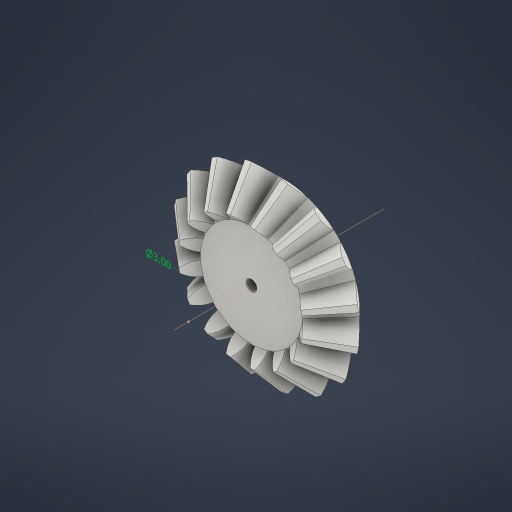
# Autodesk Inventor part: Bevel Gear2
Saved by Autodesk Inventor 2024 (Build 280153000, 153)
## iProperties
CustomPartVersion: 1
Created: 2024-03-09
Part Number: Bevel Gear2
Material: Steel, Mild
Document SubType Name: Modeling
Designer: LightStore
Categories: <?xml version="1.0" encoding="UTF-16"?> <MemberInstance><Categories><FamilyTemplate><FamilyTemplateParameter ValueType="xs:double" Id="1" ObjectReferenceKey="da_z" ObjectType="kUserParameterObject"/><FamilyTemplateParameter ValueType="xs:double" Id="2" ObjectReferenceKey="da_b" ObjectType="kUserParameterObject"/><FamilyTemplateParameter ValueType="xs:double" Id="3" ObjectReferenceKey="da_beta" ObjectType="kUserParameterObject"/><FamilyTemplateParameter ValueType="xs:double" Id="4" ObjectReferenceKey="da_dae" ObjectType="kUserParameterObject"/><FamilyTemplateParameter ValueType="xs:double" Id="5" ObjectReferenceKey="da_ve" ObjectType="kUserParameterObject"/><FamilyTemplateParameter ValueType="xs:double" Id="6" ObjectReferenceKey="da_omega" ObjectType="kUserParameterObject"/><FamilyTemplateParameter ValueType="xs:string" Id="7" ObjectReferenceKey="EAIAABAAAAAAHwAAAAAAAIAAAAAAAAAA" ObjectType="83914240" SubObjectId="SurfaceGeometry"/></FamilyTemplate><ParamToTemplateMap><ParamToTemplate CategoryParameter="//CategoryParameter[@InternalName='046C89C9-8512-4d59-83FE-43B91F4F132A']" TemplateParameter="1"/><ParamToTemplate CategoryParameter="//CategoryParameter[@InternalName='2552DF32-E462-4b46-AEBF-C6C7768E72AC']" TemplateParameter="2"/><ParamToTemplate CategoryParameter="//CategoryParameter[@InternalName='C9EE641D-15FC-4fae-A226-E94C4372FDD7']" TemplateParameter="3"/><ParamToTemplate><ParamToTemplate CategoryParameter="//CategoryParameter[@InternalName='00B6519A-459B-49c7-AD84-2E56D39A5744']" ConstantValue="-0.000000"/></ParamToTemplate><ParamToTemplate><ParamToTemplate CategoryParameter="//CategoryParameter[@InternalName='04B31F0E-C7A6-4894-AA32-9629BEFACF47']" ConstantValue="1.000000"/></ParamToTemplate><ParamToTemplate><ParamToTemplate CategoryParameter="//CategoryParameter[@InternalName='43CBEC2E-7847-49e7-A936-2F7889FCB2D9']" ConstantValue="0.200000"/></ParamToTemplate><ParamToTemplate><ParamToTemplate CategoryParameter="//CategoryParameter[@InternalName='B1EFC894-105D-4ebd-86BF-FA20ED196853']" ConstantValue="0.300000"/></ParamToTemplate><ParamToTemplate><ParamToTemplate CategoryParameter="//CategoryParameter[@InternalName='51175063-3D10-4879-93E8-6246FE8B403D']" ConstantValue="2060000000.000000"/></ParamToTemplate><ParamToTemplate><ParamToTemplate CategoryParameter="//CategoryParameter[@InternalName='A3A52E27-4454-46a9-B0BD-C932399B70AF']" ConstantValue="0.300000"/></ParamToTemplate><ParamToTemplate CategoryParameter="//CategoryParameter[@InternalName='2A200944-5A8C-41ca-B96E-8520D2E510F1']" TemplateParameter="4"/><ParamToTemplate><ParamToTemplate CategoryParameter="//CategoryParameter[@InternalName='1A637F62-92C8-44bc-B81F-10802510B579']" ConstantValue="3.484953"/></ParamToTemplate><ParamToTemplate CategoryParameter="//CategoryParameter[@InternalName='B52DD4BE-6863-48fb-BF58-89EF6F9EC65C']" TemplateParameter="5"/><ParamToTemplate><ParamToTemplate CategoryParameter="//CategoryParameter[@InternalName='3956BFF2-84D2-457d-93C2-9B0613DEBA67']" ConstantValue="1.459462"/></ParamToTemplate><ParamToTemplate CategoryParameter="//CategoryParameter[@InternalName='739CFA02-461B-4bf8-8049-181FCAD8B28F']" TemplateParameter="6"/><ParamToTemplate><ParamToTemplate CategoryParameter="//CategoryParameter[@InternalName='A27E999F-E2CE-4481-8A2A-EBF499C4C3C5']" ConstantValue="-0.000000"/></ParamToTemplate><ParamToTemplate><ParamToTemplate CategoryParameter="//CategoryParameter[@InternalName='9E1B4470-B2D3-4ff1-B813-535BB4CDF51A']" ConstantValue="3520000.000000"/></ParamToTemplate><ParamToTemplate><ParamToTemplate CategoryParameter="//CategoryParameter[@InternalName='F8452263-BFF6-458c-9FB1-07C4B99E95CD']" ConstantValue="11400000.000000"/></ParamToTemplate><ParamToTemplate><ParamToTemplate CategoryParameter="//CategoryParameter[@InternalName='3E3BB259-FD49-497f-8171-6EBC954A3479']" ConstantValue="2.000000"/></ParamToTemplate><ParamToTemplate CategoryParameter="//CategoryParameter[@InternalName='27C3BAF2-7550-4e4b-AE2C-0DB134B7D9B7']" TemplateParameter="7"/></ParamToTemplateMap><Category DisplayName="Gear" InternalName="DC85795E-93AB-48d5-8EEE-5A27447B64BD" Mnemonic="Gear"><CategoryParameter DisplayName="z" InternalName="046C89C9-8512-4d59-83FE-43B91F4F132A" Mnemonic="z"/><CategoryParameter DisplayName="b" InternalName="2552DF32-E462-4b46-AEBF-C6C7768E72AC" Mnemonic="b"/><CategoryParameter DisplayName="||b|" InternalName="C9EE641D-15FC-4fae-A226-E94C4372FDD7" Mnemonic="beta"/><CategoryParameter DisplayName="x" InternalName="00B6519A-459B-49c7-AD84-2E56D39A5744" Mnemonic="x"/><CategoryParameter DisplayName="a*" InternalName="04B31F0E-C7A6-4894-AA32-9629BEFACF47" Mnemonic="a"/><CategoryParameter DisplayName="c*" InternalName="43CBEC2E-7847-49e7-A936-2F7889FCB2D9" Mnemonic="c"/><CategoryParameter DisplayName="r|.f|*" InternalName="B1EFC894-105D-4ebd-86BF-FA20ED196853" Mnemonic="rf"/><CategoryParameter DisplayName="E" InternalName="51175063-3D10-4879-93E8-6246FE8B403D" Mnemonic="E"/><CategoryParameter DisplayName="||m|" InternalName="A3A52E27-4454-46a9-B0BD-C932399B70AF" Mnemonic="mi"/><Category DisplayName="BevelGear" InternalName="0C98F69A-0C2B-4791-B2FE-7691BB227E77" Mnemonic="BevelGear"><CategoryParameter DisplayName="d|.ae|" InternalName="2A200944-5A8C-41ca-B96E-8520D2E510F1" Mnemonic="dae"/><CategoryParameter DisplayName="d|.ai|" InternalName="1A637F62-92C8-44bc-B81F-10802510B579" Mnemonic="dai"/><CategoryParameter DisplayName="A|.e|" InternalName="B52DD4BE-6863-48fb-BF58-89EF6F9EC65C" Mnemonic="ve"/><CategoryParameter DisplayName="A|.i|" InternalName="3956BFF2-84D2-457d-93C2-9B0613DEBA67" Mnemonic="vi"/><CategoryParameter DisplayName="||S|" InternalName="739CFA02-461B-4bf8-8049-181FCAD8B28F" Mnemonic="omega"/><CategoryParameter DisplayName="x|.t|" InternalName="A27E999F-E2CE-4481-8A2A-EBF499C4C3C5" Mnemonic="xt"/><CategoryParameter DisplayName="||s||.Flim|" InternalName="9E1B4470-B2D3-4ff1-B813-535BB4CDF51A" Mnemonic="sFlim"/><CategoryParameter DisplayName="||s||.Hlim|" InternalName="F8452263-BFF6-458c-9FB1-07C4B99E95CD" Mnemonic="sHlim"/><CategoryParameter DisplayName="type" InternalName="3E3BB259-FD49-497f-8171-6EBC954A3479" Mnemonic="type"/><CategoryParameter DisplayName="PitchDiameter" InternalName="27C3BAF2-7550-4e4b-AE2C-0DB134B7D9B7" Mnemonic="IDS_PITCHDIAM"/></Category></Category></Categories></MemberInstance>
Mass: 60.9118 g
Surface Area: 34.3074 cm^2
Volume: 7.7496 cm^3
Density: 7.86 g/cm^3
Appearance: Steel
Author: LightStore
Autodesk Inventor part; units mm, degrees
ref_plane "Mesh Plane2" through (0, 0, 0) normal (0.9807853, 0.1950903, 0) x (0, 0, 1)
sketch "Teeth Body Sketch" plane through (0, 0, 0) normal (1, 0, 0) x (0, 1, 0)
  line L0 (0, 0) -> (21.454416, -26.545584) construction
  line L1 (21.454416, -26.545584) -> (26.12132, -21.87868)
  line L2 (26.12132, -21.87868) -> (0, 0) construction
  line L3 (24, -24) -> (0, 0) construction
  line L4 (14.311609, -17.707778) -> (17.424764, -14.594623)
  line L5 (21.454416, -26.545584) -> (14.311609, -17.707778)
  line L6 (26.12132, -21.87868) -> (17.424764, -14.594623)
  line L7 (0, -39.386751) -> (0, 6.564458)
  line L8 (0, -24) -> (26.12132, -24) construction
  dimension "d0" = 48
  dimension "d1" = 42.90883
  dimension "d2" = 52.24264
  dimension "d3" = 11.3
  dimension "d4" = 21.87868
  constraints: 16 end point, 4 point on line, 3 perpendicular, 2 collinear, 1 horizontal alignment, 1 vertical alignment
  measures "d0" diameter of L3.start L7
  measures "d1" diameter of L0.end L7
  measures "d2" diameter of L1.end L7
  measures "d3" distance between parallel lines of L1 L4
  measures "d4" vertical distance of L1.end L0.start
revolve "Teeth Body" add sketch "Teeth Body Sketch" angle 360 about axis through (0, 0, 0) along (0, 0, 1)
ref_plane "Tooth Plane" through (0, 24, -24) normal (0, -0.7071068, 0.7071068) x (1, 0, 0)
sketch "Start Sketch" plane through (0, 24, -24) normal (0, -0.7071068, 0.7071068) x (1, 0, 0)
  line L0 (0, -23.505131) -> (0, 10.644758)
  arc A0 (-1.269242, -4.392) -> (-5.97451, 4.518714) centre (-13.855964, -5.340713) ccw
  arc A1 (5.97451, 4.518714) -> (1.269242, -4.392) centre (13.855964, -5.340713) ccw
  line L1 (-1.269242, -4.392) -> (1.269242, -4.392)
  arc A2 (5.97451, 4.518714) -> (-5.97451, 4.518714) centre (0, -33.941125) ccw
  dimension "d7" = 12.62242
  dimension "d8" = 13.85596
  dimension "d9" = 28.60041
  dimension "d57" = 38.92113
  dimension "d58" = 29.54913
  constraints: 6 point on circle, 3 centre point, 3 symmetric about line, 2 end point, 1 coincident, 1 perpendicular, 1 other
  measures "d7" radius of A0
  measures "d8" horizontal distance of point (0, -33.941) A0.centre
  measures "d9" vertical distance of point (0, -33.941) A0.centre
  measures "d57" radius of A2
  measures "d58" distance from line of A2.centre L1
sketch "End Sketch" plane through (0, 15.776348, -15.776348) normal (0, -0.7071068, 0.7071068) x (1, 0, 0)
  line L0 (0, -15.35404) -> (0, 6.953444)
  arc A0 (-0.834334, -2.887072) -> (-3.927331, 2.970367) centre (-9.108188, -3.510706) ccw
  arc A1 (3.927331, 2.970367) -> (0.834334, -2.887072) centre (9.108188, -3.510706) ccw
  line L1 (-0.834334, -2.887072) -> (0.834334, -2.887072)
  arc A2 (3.927331, 2.970367) -> (-3.927331, 2.970367) centre (0, -22.311125) ccw
  dimension "d12" = 8.29732
  dimension "d15" = 9.10819
  dimension "d16" = 18.80042
  dimension "d59" = 25.58472
  dimension "d60" = 19.42405
  constraints: 6 point on circle, 3 centre point, 3 symmetric about line, 2 end point, 1 coincident, 1 other
  measures "d12" radius of A0
  measures "d15" horizontal distance of A0.centre point (0, -22.311)
  measures "d16" vertical distance of A0.centre point (0, -22.311)
  measures "d59" radius of A2
  measures "d60" distance from line of A2.centre L1
loft "Loft" cut profiles "Start Sketch", "End Sketch"
pattern_circular "Circular Pattern" count 16 over 360 about axis through (0, 0, 0) along (0, 0, 1) of "Loft"
ref_plane "End Plane" through (0, 15.776348, -15.776348) normal (0, -0.7071068, 0.7071068) x (1, 0, 0)
sketch3d "3D Sketch Right"
ref_plane "End Plane Right" through (-3.313379, 15.424483, -15.776348) normal (0.1485079, -0.6913359, 0.7071068) x (0.9776967, 0.210022, 0)
sketch "End Sketch Right" plane through (-3.313379, 15.424483, -15.776348) normal (0.1485079, -0.6913359, 0.7071068) x (0.9776967, 0.210022, 0)
  arc A0 (-0.834334, -2.887072) -> (-3.927331, 2.970367) centre (-9.108188, -3.510706) ccw
  line L0 (0, -30.205233) -> (0, 11.660762)
  arc A1 (3.927331, 2.970367) -> (0.834334, -2.887072) centre (9.108188, -3.510706) ccw
  line L1 (-0.834334, -2.887072) -> (0.834334, -2.887072)
  arc A2 (3.927331, 2.970367) -> (-3.927331, 2.970367) centre (0, -22.311125) ccw
  dimension "d70" = 9.10819
  dimension "d71" = 18.80042
  dimension "d72" = 8.29732
  dimension "d73" = 19.42405
  dimension "d74" = 25.58472
  constraints: 6 point on circle, 3 centre point, 3 symmetric about line, 2 end point, 1 coincident, 1 perpendicular, 1 other
  measures "d70" horizontal distance of A2.centre A0.centre
  measures "d71" vertical distance of point (0, -22.311) A0.centre
  measures "d72" radius of A0
  measures "d73" distance from line of point (0, -22.311) L1
  measures "d74" radius of A2
feature "Loft Right" [suppressed]
pattern_circular "Circular Pattern Right" [suppressed]
sketch3d "3D Sketch Left"
ref_plane "End Plane Left" through (3.335768, 15.424483, -15.785404) normal (-0.1494462, -0.6910343, 0.707204) x (0.9774044, -0.2113779, 0)
sketch "End Sketch Left" plane through (3.335768, 15.424483, -15.785404) normal (-0.1494462, -0.6910343, 0.707204) x (0.9774044, -0.2113779, 0)
  line L0 (0, -32.902845) -> (0, 14.363747)
  arc A0 (-0.834334, -2.884005) -> (-3.927331, 2.973434) centre (-9.108188, -3.507639) ccw
  arc A1 (3.927331, 2.973434) -> (0.834334, -2.884005) centre (9.108188, -3.507639) ccw
  line L1 (-0.834334, -2.884005) -> (0.834334, -2.884005)
  ellipse E0 centre (0, -10.318538) end of major axis (17.424764, -10.318538) minor radius 12.322862
  arc A2 (3.927331, 2.973434) -> (-3.927331, 2.973434) centre (0, -22.308059) ccw
  dimension "d56" = 12.32286
  dimension "d30" = 8.29732
  dimension "d31" = 9.10819
  dimension "d32" = 18.80042
  dimension "d61" = 25.58472
  dimension "d62" = 19.42405
  constraints: 6 point on circle, 3 centre point, 3 symmetric about line, 2 end point, 1 coincident, 2 other
  measures "d30" radius of A0
  measures "d31" horizontal distance of point (0, -22.308) A0.centre
  measures "d32" vertical distance of A0.centre point (0, -22.308)
  measures "d61" radius of A2
  measures "d62" distance from line of point (0, -22.308) L1
feature "Loft Left" [suppressed]
pattern_circular "Circular Pattern Left" [suppressed]
sketch "Body Sketch" plane through (0, 0, 0) normal (1, 0, 0) x (0, 1, 0)
  line L0 (0, -35.037536) -> (0, -19.530831)
  line L1 (21.454416, -26.545584) -> (14.311609, -17.707778)
  line L2 (14.311609, -17.707778) -> (0, -17.707778)
  line L3 (21.454416, -26.545584) -> (0, -26.545584)
  constraints: 4 end point, 2 perpendicular, 2 point on line
sketch "Body Sketch outline for Fix Body" plane through (0, 0, 0) normal (1, 0, 0) x (0, 1, 0)
  line L0 (0, -26.545584) -> (21.454416, -26.545584)
  line L1 (0, -17.707778) -> (0, -26.545584)
  line L2 (14.311609, -17.707778) -> (0, -17.707778)
  line L3 (21.454416, -26.545584) -> (14.311609, -17.707778)
revolve "Fix Body" add sketch "Body Sketch outline for Fix Body" angle 360 about axis through (0, 0, 0) along (0, 0, 1)
sketch "Sketch6" plane through (0, 0, 0) normal (1, 0, 0) x (0, 1, 0)
  line L0 (24, -24) -> (0, 0)
  line L1 (0, -37.799919) -> (0, 6.299986)
surface revolve "Pitch Diameter" sketch "Sketch6" angle 360 about axis through (0, 0, 0) along (0, 0, 1) shown no curves L0
sketch "Sketch8" plane through (0, 0, -26.545584) normal (0, 0, -1) x (-1, 0, 0)
  point P0 (0, 0)
ref_plane "Work Plane6" through (0, 0.035237, -26.545584) normal (0, 0, -1) x (-1, 0, 0)
sketch "Sketch12" plane through (0, 0, -26.545584) normal (0, 0, -1) x (-1, 0, 0)
  circle A0 centre (0, 0) radius 1.5
  dimension "d113" = 3
  constraints: 1 centre point, 1 coincident
  measures "d113" diameter of A0
extrude "Extrusion6" cut sketch "Sketch12" against normal blind 20
thread "Thread1" size "M3x0.5" class "6H" standard "ANSI Metric M Profile" length 4000
equation "\"d0\" = da_de"
equation "\"d1\" = da_dfe"
equation "\"d2\" = da_dae"
equation "\"d3\" = da_b"
equation "\"d4\" = da_ve"
equation "\"d7\" = fd_rr"
equation "\"d8\" = fd_x"
equation "\"d9\" = fd_y"
equation "\"d57\" = 0.5 * fd_dva + 0.3 * da_he"
equation "\"d58\" = 0.5 * fd_dva - 1.12 * da_he"
equation "\"da_teethtype\" = 0"
equation "\"da_b\" = 11.3"
equation "\"da_de\" = 48"
equation "\"da_dae\" = 52.24264"
equation "\"da_dfe\" = 42.90883"
equation "\"da_le\" = 33.94113"
equation "\"da_omega\" = 90deg"
equation "\"da_beta\" = 0"
equation "\"da_delta\" = 45deg"
equation "\"da_alpha\" = 20deg"
equation "\"da_he\" = 6.6"
equation "\"da_ve\" = 21.87868"
equation "\"da_zv\" = 22.627417"
equation "\"fd_loft\" = da_b + 0.05 * da_he"
equation "\"fd_x\" = fd_x1 + fd_x2"
equation "\"fd_y\" = fd_y1 - fd_y2"
equation "\"fd_dd\" = fd_dva - 0.8 * da_he"
equation "\"da_dvw\" = 67.88225"
equation "\"d11\" = fd_loft"
equation "\"da_dm\" = 40.00969"
equation "\"da_x\" = 0"
equation "\"da_m\" = 3"
equation "\"d50\" = da_omega"
equation "\"fd_rr\" = 12.622425"
equation "\"fd_dva\" = 73.882251"
equation "\"fd_x1\" = 2.380419"
equation "\"fd_x2\" = 11.475545"
equation "\"fd_y1\" = 33.857549"
equation "\"fd_y2\" = 5.257136"
body "Solid1"
body "Srf1"
